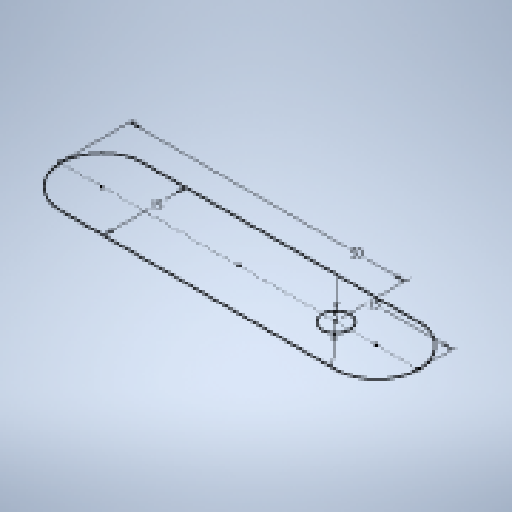
# Autodesk Inventor part: Arm_3
Saved by Autodesk Inventor 2023 (Build 270158000, 158)
## iProperties
Created: 2022-04-08
Part Number: Arm_3
Material: 一般
Document SubType Name: Modeling
Designer: device
Density: 1 g/cm^3
Appearance: 預設
Author: device
Autodesk Inventor part; units mm, degrees
ref_plane "YZ Plane" through (0, 0, 0) normal (1, 0, 0) x (0, 1, 0)
ref_plane "XZ Plane" through (0, 0, 0) normal (0, 1, 0) x (-1, 0, 0)
ref_plane "XY Plane" through (0, 0, 0) normal (0, 0, 1) x (1, 0, 0)
sketch "草圖1" plane through (0, 0, 0) normal (0, 1, 0) x (-1, 0, 0)
  circle A0 centre (0, 0) radius 2.5
  line L0 (-15, 0) -> (60, 0) construction
  line L1 (-7.5, 7.5) -> (52.5, 7.5)
  line L2 (52.5, -7.5) -> (-7.5, -7.5)
  arc A1 (-7.5, 7.5) -> (-7.5, -7.5) centre (-7.5, 0) ccw
  arc A2 (52.5, -7.5) -> (52.5, 7.5) centre (52.5, 0) ccw
  line L3 (52.5, -7.5) -> (60, -7.5)
  line L4 (60, -7.5) -> (60, 7.5)
  line L5 (60, 7.5) -> (52.5, 7.5)
  line L6 (52.5, 7.5) -> (52.5, -7.5)
  point P0 (22.5, 0)
  point P1 (60, 0)
  point P2 (-15, 0)
  point P3 (60, 0)
  dimension "d0" = 5
  dimension "d5" = 15
  dimension "d6" = 60
  dimension "d7" = 15
  constraints: 16 end point, 8 point on circle, 5 tangent, 3 centre point, 3 parallel, 3 point on line, 2 horizontal, 1 coincident, 1 midpoint, 1 perpendicular
  measures "d0" diameter of A0
  measures "d5" distance between parallel lines of L1 L2
  measures "d6" distance of point (0, 0) point (60, 0)
  measures "d7" distance of point (0, 0) point (-15, 0)
extrude "擠出1" add sketch "草圖1" along normal mid plane 3
sketch "草圖2" plane through (0, 1.5, 0) normal (0, 1, 0) x (1, 0, 0)
  arc A0 (7.5, -7.5) -> (7.5, 7.5) centre (7.5, 0) ccw construction
  circle A1 centre (0, 0) radius 2.5 construction
  line L0 (-55.5, 12) -> (-52.5, 12)
  line L1 (-52.5, 12) -> (-52.5, -24)
  line L2 (-52.5, -24) -> (-55.5, -24)
  line L3 (-55.5, -24) -> (-55.5, 12)
  line L4 (-55.5, 6) -> (-52.5, 6)
  line L5 (-52.5, 6) -> (-52.5, -18)
  line L6 (-52.5, -18) -> (-55.5, -18)
  line L7 (-55.5, -18) -> (-55.5, 6)
  line L8 (-75, 0) -> (30, 0) construction
  line L9 (-60, -7.5) -> (7.5, -7.5) projected
  line L10 (7.5, 7.5) -> (-60, 7.5) projected
  line L11 (-60, 7.5) -> (-60, -7.5) projected
  point P0 (-52.5, -6)
  point P1 (-54, -18)
  point P2 (-54, 6)
  dimension "d10" = 36
  dimension "d11" = 3
  dimension "d12" = 24
  dimension "d14" = 6
  dimension "d32" = 4.5
  constraints: 16 end point, 4 midpoint, 4 parallel, 2 horizontal, 2 perpendicular, 2 point on line
  measures "d10" distance of L0.end L1.end
  measures "d11" distance of L0.start L0.end
  measures "d12" distance of point (-54, -18) point (-54, 6)
  measures "d14" distance from line of L8 point (-54, 6)
  measures "d32" distance between parallel lines of L11 L3
extrude "擠出2" add sketch "草圖2" along normal blind 12.5 and the other way blind 6 contours L0 L1 L10 L3 | L10 L1 L4 L3 | L4 L1 L9 L3 | L9 L1 L6 L3 | L6 L1 L2 L3
sketch "草圖3" plane through (-52.5, -4.5, -12) normal (1, 0, 0) x (0, 0, -1)
  line L0 (0, 0) -> (0, 18.5) projected
  line L1 (-36, 18.5) -> (0, 18.5) projected
  line L2 (-36, 18.5) -> (-36, 0) projected
  line L3 (0, 0) -> (-36, 0) projected
  line L4 (-19.5, 3) -> (-4.5, 3) projected
  line L5 (-19.5, 6) -> (-19.5, 3) projected
  line L6 (-4.5, 6) -> (-19.5, 6) projected
  line L7 (-4.5, 3) -> (-4.5, 6) projected
  line L8 (0, 18.5) -> (-36, 18.5) projected
  line L9 (-30, 18.5) -> (-6, 18.5)
  line L10 (-6, 18.5) -> (-6, 6)
  line L11 (-6, 6) -> (-30, 6)
  line L12 (-30, 6) -> (-30, 18.5)
  point P0 (-12, 4.5)
  point P1 (-18, 18.5)
  point P2 (-19.5, 6)
  point P3 (-6, 18.5)
  dimension "d19" = 24
  dimension "d20" = 12.5
  constraints: 8 end point, 2 midpoint, 2 parallel, 1 horizontal, 1 perpendicular, 1 point on line
  measures "d19" distance of L10.end L11.end
  measures "d20" distance of L9.end L10.end
extrude "擠出3" cut sketch "草圖3" against normal up to surface (3 mm away) contours L10 L6 L11 L12 L1
sketch "草圖4" plane through (-52.5, -4.5, 24) normal (1, 0, 0) x (0, 0, -1)
  line L0 (6, 6) -> (6, 18.5) construction
  line L1 (0, 18.5) -> (6, 18.5) construction
  line L2 (0, 18.5) -> (0, 0) construction
  line L3 (36, 0) -> (0, 0) construction
  line L4 (36, 0) -> (36, 18.5) construction
  line L5 (30, 18.5) -> (36, 18.5) construction
  line L6 (30, 18.5) -> (30, 6) construction
  line L7 (31.5, 6) -> (30, 6) construction
  line L8 (31.5, 3) -> (31.5, 6) construction
  line L9 (16.5, 3) -> (31.5, 3) construction
  line L10 (16.5, 6) -> (16.5, 3) construction
  line L11 (16.5, 6) -> (6, 6) construction
  line L12 (0, 0) -> (0, 18.5) construction
  line L13 (0, 12.25) -> (36, 12.25) construction
  line L14 (36, 0) -> (36, 18.5) construction
  circle A0 centre (3.5, 12.25) radius 1.25
  circle A1 centre (32.5, 12.25) radius 1.25
  line L15 (18, 12.25) -> (18, 14.7148) construction
  point P0 (24, 4.5)
  point P1 (6, 12.25)
  dimension "d23" = 2.5
  dimension "d24" = 29
  constraints: 5 point on line, 4 end point, 2 centre point, 2 midpoint, 1 equal radius, 1 perpendicular, 1 vertical, 1 other
  measures "d23" diameter of A0
  measures "d24" distance of A1.centre A0.centre
extrude "擠出4" cut sketch "草圖4" against normal up to surface (3 mm away)
sketch "草圖5" plane through (0, 1.5, 0) normal (0, 1, 0) x (1, 0, 0)
  line L0 (-52.5, 12) -> (-52.5, -24) construction
  line L1 (-52.5, -24) -> (-55.5, -24) construction
  line L2 (-55.5, -24) -> (-55.5, 12) construction
  line L3 (-55.5, 12) -> (-52.5, 12) construction
  line L4 (-49.5, -10.5) -> (-52.5, -10.5)
  line L5 (-58.5, -10.5) -> (-58.5, -7.5)
  line L6 (-58.5, -4.5) -> (-55.5, -4.5)
  line L7 (-49.5, -4.5) -> (-49.5, -7.5)
  line L8 (-52.5, -4.5) -> (-49.5, -4.5)
  line L9 (-55.5, -4.5) -> (-52.5, -4.5)
  line L10 (-49.5, -7.5) -> (-49.5, -10.5)
  line L11 (-58.5, -7.5) -> (-58.5, -4.5)
  line L12 (-52.5, -10.5) -> (-55.5, -10.5)
  line L13 (-55.5, -10.5) -> (-58.5, -10.5)
  line L14 (-52.5, -10.5) -> (-55.5, -10.5)
  line L15 (-55.5, -10.5) -> (-55.5, -7.5)
  line L16 (-55.5, -7.5) -> (-52.5, -7.5)
  line L17 (-52.5, -7.5) -> (-52.5, -10.5)
  point P0 (0, 0)
  point P1 (-55.5, -10.5)
  constraints: 28 end point, 15 parallel, 7 perpendicular, 4 equal length, 4 horizontal, 4 point on line
extrude "擠出5" cut sketch "草圖5" against normal blind 3 contours L4 L17 L16 L15 L13 L5 L11 L6 L9 L8 L7 L10
extrude "擠出6" add sketch "草圖5" against normal blind 3 separate body contours L4 L17 L16 L15 L13 L5 L11 L6 L9 L8 L7 L10
mirror "鏡射1" about plane through (0, 0, 0) normal (0, 0, 1) of "擠出5" bodies 1
mirror "鏡射2" about plane through (0, 0, 0) normal (0, 0, 1) of "擠出6" bodies 2
